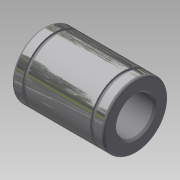
# Autodesk Inventor part: U-LMU0 50
Saved by Autodesk Inventor 2020.1 (Build 241239000, 239)
## iProperties
Created: 2019-12-03
Part Number: U-LMU0 50
Material: Generic
Catalog Web Link: https://us.misumi-ec.com/vona2/detail/110302150430/?HissuCode=U-LMU0.50&searchFlow=results2similartn&curSearch=%7b%22field%22%3a%22%40search%22%2c%22seriesCode%22%3a%22110302150430%22%2c%22innerCode%22%3a%22%22%2c%22sort%22%3a1%2c%22specSortFlag%22%3a0%2c%22allSpecFlag%22%3a0%2c%22page%22%3a1%2c%22pageSize%22%3a%2260%22%2c%2200000043049%22%3a%22mig00000001470339%22%2c%2200000043050%22%3a%22mig00000001470340%22%2c%2200000043048%22%3a%22mig00000001470341%22%2c%2200000028976%22%3a%22mig00000001470355%22%2c%22fixedInfo%22%3a%22MDM0000198303811030215043011%7c19%22%7d&Tab=preview
Description: U-LMU-Linear Bushings - Single Bushing
Vendor: MISUMI
Document SubType Name: Modeling
Designer: Autodesk Inc.
Manufacturer: MISUMI
Mass: 8.15316 g
Surface Area: 41.0689 cm^2
Volume: 8.15316 cm^3
Density: 1 g/cm^3
Appearance: PSOLRGB-175-175-175
Category: FIRSTChoice
Company: Autodesk Inc.
PSOL_IDENT_0: {$CADENAS_DATA\23d-libs\misumi\inch\linear_motion\bushings\u_lmu.prj},157 {VTYP=3D},{NB=U-LMU0.50},{
PSOL_IDENT_1: LINA=U-LMU0.50},{NN=U-LMU},{DATE=05.01.2018 04:43:42},{GEOMDATE=05.01.2018 04:43:42},{VERSION=},{LIN
PSOL_IDENT_2: EID=30},{WBVAR=},{WBNUMERIC=}  {NB=U-LMU0.50},{LINA=U-LMU0.50},{KT=DUMMY},{PN=U-LMU0.50},{TYPE=U-LMU
PSOL_IDENT_3: },{MATOC=52100 Bearing Steel},{HARD=58HRC~},{MATB=52100 Bearing Steel},{MATC=Plastic (Delrin Class)}
PSOL_IDENT_4: ,{TEMP=-4 - 176°F},{MATS=NBR (Nitrile Rubber)},{DR=0.50},{DRNOM=1/2},{DRTOLMAX=0.4997},{DRTOLMIN=0.4
PSOL_IDENT_5: 993},{DR0=0.500},{DNOM=7/8},{DTOLMAX=0.8750},{DTOLMIN=0.8746},{D0=0.8750},{LNOM=1-1/4},{L0=1.250},{B
PSOL_IDENT_6: NOM=7/8},{B0=0.875},{W=0.046},{D1=0.821},{R=0.030},{LCD=96},{LCS=107},{MASS=1.36}
NN: U-LMU
NT: Linear Bushings - Single Bushing
NB: U-LMU0.50
NBSYN: $PN.
LINA: U-LMU0.50
PN: U-LMU0.50
MATOC: 52100 Bearing Steel
MATB: 52100 Bearing Steel
MATC: Plastic (Delrin Class)
MATS: NBR (Nitrile Rubber)
DRNOM: 1/2
DRTOLMAX: 0.4997
DRTOLMIN: 0.4993
DNOM: 7/8
DTOLMAX: 0.875
DTOLMIN: 0.8746
LNOM: 1-1/4
BNOM: 7/8
W: 0.046
D1: 0.821
LCD: 96
LCS: 107
MASS: 1.36
SUPPLIER: MISUMI
ARTICLENO: U-LMU0.50
BOMINFO: U-LMU0.50
CREATOR: CADENAS GmbH
Author: Autodesk Inc.
Comments: Linear Bushings - Single Bushing
Autodesk Inventor part; units mm, degrees
ref_plane "YZ Plane" through (0, 0, 0) normal (1, 0, 0) x (0, 1, 0)
ref_plane "XZ Plane" through (0, 0, 0) normal (0, 1, 0) x (-1, 0, 0)
ref_plane "XY Plane" through (0, 0, 0) normal (0, 0, 1) x (1, 0, 0)
sketch "Sketch_1" plane through (0, 0, 0) normal (0, 0, 1) x (1, 0, 0)
  line L0 (31.75, 0) -> (0, 0)
  line L1 (0, 6.985) -> (0.635, 6.35)
  line L2 (0.635, 6.35) -> (31.115, 6.35)
  line L3 (31.115, 6.35) -> (31.75, 6.985)
  line L4 (31.75, 6.985) -> (31.75, 10.3505)
  arc A0 (31.75, 10.3505) -> (30.988, 11.1125) centre (30.988, 10.3505) ccw
  line L5 (30.988, 11.1125) -> (28.1559, 11.1125)
  line L6 (28.1559, 11.1125) -> (28.1559, 10.4267)
  line L7 (28.1559, 10.4267) -> (26.9875, 10.4267)
  line L8 (26.9875, 10.4267) -> (26.9875, 11.1125)
  line L9 (26.9875, 11.1125) -> (4.7625, 11.1125)
  line L10 (4.7625, 11.1125) -> (4.7625, 10.4267)
  line L11 (4.7625, 10.4267) -> (3.5941, 10.4267)
  line L12 (3.5941, 10.4267) -> (3.5941, 11.1125)
  line L13 (3.5941, 11.1125) -> (0.762, 11.1125)
  arc A1 (0.762, 11.1125) -> (0, 10.3505) centre (0.762, 10.3505) ccw
  line L14 (0, 10.3505) -> (0, 6.985)
  constraints: 30 end point, 4 point on circle, 2 centre point
revolve "Revolution1" add sketch "Sketch_1" angle 360 about axis through (31.75, 0, 0) along (1, 0, 0)
body "Solid1"
